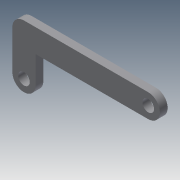
# Autodesk Inventor part: neco5
Saved by Autodesk Inventor 2013 (Build 170138000, 138)
## iProperties
Created: 2013-03-09
Part Number: neco5
Material: Generic
Document SubType Name: Modeling
Designer: idle-rug
Density: 1 g/cm^3
Author: idle-rug
Autodesk Inventor part; units mm, degrees
ref_plane "YZ Plane" through (0, 0, 0) normal (1, 0, 0) x (0, 1, 0)
ref_plane "XZ Plane" through (0, 0, 0) normal (0, 1, 0) x (-1, 0, 0)
ref_plane "XY Plane" through (0, 0, 0) normal (0, 0, 1) x (1, 0, 0)
sketch "Sketch1" plane through (0, 0, 0) normal (0, 1, 0) x (-1, 0, 0)
  line L0 (-16, -3) -> (16, -3)
  line L1 (16, -3) -> (16, 3)
  line L2 (16, 3) -> (-16, 3)
  line L3 (-16, 3) -> (-16, -3)
  line L4 (-16, -3) -> (16, 3) construction
  line L5 (16, -3) -> (-16, 3) construction
  circle A0 centre (16, 0) radius 3
  circle A1 centre (-16, 0) radius 3
  line L6 (16, 0) -> (16, -10)
  circle A2 centre (16, -10) radius 3
  line L7 (19, 0) -> (19, -10)
  line L8 (19, -10) -> (13, -10)
  line L9 (13, -10) -> (13, 0)
  line L10 (13, 0) -> (19, 0)
  point P0 (0, 0)
  dimension "d0" = 32
  dimension "d1" = 6
  dimension "d2" = 6
  dimension "d3" = 6
  dimension "d4" = 10
  dimension "d5" = 6
  constraints: 22 end point, 4 midpoint, 4 point on circle, 3 centre point, 3 parallel, 3 tangent, 2 perpendicular, 1 coincident, 1 horizontal
  measures "d0" distance of L2.end L1.end
  measures "d1" distance of L1.end L0.end
  measures "d2" diameter of A0
  measures "d3" diameter of A1
  measures "d4" distance of L6.start L6.end
  measures "d5" diameter of A2
extrude "Extrusion1" add sketch "Sketch1" along normal blind 2
sketch "Sketch2" plane through (0, 2, 0) normal (0, 1, 0) x (1, 0, 0)
  arc A0 (16, -3) -> (16, 3) centre (16, 0) ccw projected
  arc A1 (-13, 10) -> (-19, 10) centre (-16, 10) ccw projected
  circle A2 centre (-16, 10) radius 1.5
  circle A3 centre (16, 0) radius 1.5
  point P0 (0, 0)
  dimension "d8" = 3
  dimension "d9" = 3
  constraints: 2 centre point, 2 coincident
  measures "d8" diameter of A2
  measures "d9" diameter of A3
extrude "Extrusion2" cut sketch "Sketch2" against normal blind 2
body "Solid1"
